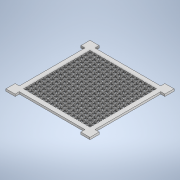
# Autodesk Inventor part: LED_Abstand
Saved by Autodesk Inventor 2022 (Build 260153000, 153)
## iProperties
Created: 2022-02-17
Part Number: LED_Abstand
Material: Generisch
Document SubType Name: Modeling
Designer: Max
Density: 1 g/cm^3
Appearance: Vorgabe
Author: Max
Autodesk Inventor part; units mm, degrees
(part 1 of 3)
ref_plane "YZ Plane" through (0, 0, 0) normal (1, 0, 0) x (0, 1, 0)
ref_plane "XZ Plane" through (0, 0, 0) normal (0, 1, 0) x (-1, 0, 0)
ref_plane "XY Plane" through (0, 0, 0) normal (0, 0, 1) x (1, 0, 0)
sketch "Skizze1" plane through (0, 0, 0) normal (0, 1, 0) x (-1, 0, 0)
  line L0 (-21.9, -21.9) -> (-28.1, -21.9)
  line L1 (-28.1, -21.9) -> (-28.1, -28.1)
  line L2 (-28.1, -28.1) -> (-21.9, -28.1)
  line L3 (-21.9, -28.1) -> (-21.9, -21.9)
  line L4 (-21.9, -31.9) -> (-28.1, -31.9)
  line L5 (-28.1, -31.9) -> (-28.1, -38.1)
  line L6 (-28.1, -38.1) -> (-21.9, -38.1)
  line L7 (-21.9, -38.1) -> (-21.9, -31.9)
  line L8 (-21.9, -41.9) -> (-28.1, -41.9)
  line L9 (-28.1, -41.9) -> (-28.1, -48.1)
  line L10 (-28.1, -48.1) -> (-21.9, -48.1)
  line L11 (-21.9, -48.1) -> (-21.9, -41.9)
  line L12 (-21.9, -51.9) -> (-28.1, -51.9)
  line L13 (-28.1, -51.9) -> (-28.1, -58.1)
  line L14 (-28.1, -58.1) -> (-21.9, -58.1)
  line L15 (-21.9, -58.1) -> (-21.9, -51.9)
  line L16 (-21.9, -61.9) -> (-28.1, -61.9)
  line L17 (-28.1, -61.9) -> (-28.1, -68.1)
  line L18 (-28.1, -68.1) -> (-21.9, -68.1)
  line L19 (-21.9, -68.1) -> (-21.9, -61.9)
  line L20 (-21.9, -28.1) -> (-21.9, -31.9) construction
  line L21 (-21.9, -38.1) -> (-21.9, -41.9) construction
  line L22 (-21.9, -48.1) -> (-21.9, -51.9) construction
  line L23 (-21.9, -58.1) -> (-21.9, -61.9) construction
  line L24 (-21.9, -21.9) -> (-21.9, -10) construction
  line L25 (-21.9, -21.9) -> (-10, -21.9) construction
  line L26 (-21.9, -71.9) -> (-28.1, -71.9)
  line L27 (-28.1, -71.9) -> (-28.1, -78.1)
  line L28 (-28.1, -78.1) -> (-21.9, -78.1)
  line L29 (-21.9, -78.1) -> (-21.9, -71.9)
  line L30 (-21.9, -81.9) -> (-28.1, -81.9)
  line L31 (-28.1, -81.9) -> (-28.1, -88.1)
  line L32 (-28.1, -88.1) -> (-21.9, -88.1)
  line L33 (-21.9, -88.1) -> (-21.9, -81.9)
  line L34 (-21.9, -91.9) -> (-28.1, -91.9)
  line L35 (-28.1, -91.9) -> (-28.1, -98.1)
  line L36 (-28.1, -98.1) -> (-21.9, -98.1)
  line L37 (-21.9, -98.1) -> (-21.9, -91.9)
  line L38 (-21.9, -101.9) -> (-28.1, -101.9)
  line L39 (-28.1, -101.9) -> (-28.1, -108.1)
  line L40 (-28.1, -108.1) -> (-21.9, -108.1)
  line L41 (-21.9, -108.1) -> (-21.9, -101.9)
  line L42 (-21.9, -111.9) -> (-28.1, -111.9)
  line L43 (-28.1, -111.9) -> (-28.1, -118.1)
  line L44 (-28.1, -118.1) -> (-21.9, -118.1)
  line L45 (-21.9, -118.1) -> (-21.9, -111.9)
  line L46 (-21.9, -78.1) -> (-21.9, -81.9) construction
  line L47 (-21.9, -88.1) -> (-21.9, -91.9) construction
  line L48 (-21.9, -98.1) -> (-21.9, -101.9) construction
  line L49 (-21.9, -108.1) -> (-21.9, -111.9) construction
  line L50 (-21.9, -68.1) -> (-21.9, -71.9) construction
  line L51 (-21.9, -121.9) -> (-28.1, -121.9)
  line L52 (-28.1, -121.9) -> (-28.1, -128.1)
  line L53 (-28.1, -128.1) -> (-21.9, -128.1)
  line L54 (-21.9, -128.1) -> (-21.9, -121.9)
  line L55 (-21.9, -131.9) -> (-28.1, -131.9)
  line L56 (-28.1, -131.9) -> (-28.1, -138.1)
  line L57 (-28.1, -138.1) -> (-21.9, -138.1)
  line L58 (-21.9, -138.1) -> (-21.9, -131.9)
  line L59 (-21.9, -141.9) -> (-28.1, -141.9)
  line L60 (-28.1, -141.9) -> (-28.1, -148.1)
  line L61 (-28.1, -148.1) -> (-21.9, -148.1)
  line L62 (-21.9, -148.1) -> (-21.9, -141.9)
  line L63 (-21.9, -151.9) -> (-28.1, -151.9)
  line L64 (-21.9, -138.1) -> (-21.9, -141.9) construction
  line L65 (-21.9, -148.1) -> (-21.9, -151.9) construction
  line L66 (-28.1, -151.9) -> (-28.1, -158.1)
  line L67 (-21.9, -158.1) -> (-21.9, -151.9)
  line L68 (-28.1, -158.1) -> (-21.9, -158.1)
  line L69 (-21.9, -128.1) -> (-21.9, -131.9) construction
  line L70 (-28.1, -178.1) -> (-21.9, -178.1)
  line L71 (-21.9, -171.9) -> (-28.1, -171.9)
  line L72 (-28.1, -171.9) -> (-28.1, -178.1)
  line L73 (-21.9, -178.1) -> (-21.9, -171.9)
  line L74 (-28.1, -168.1) -> (-21.9, -168.1)
  line L75 (-21.9, -168.1) -> (-21.9, -171.9) construction
  line L76 (-21.9, -161.9) -> (-28.1, -161.9)
  line L77 (-28.1, -161.9) -> (-28.1, -168.1)
  line L78 (-21.9, -168.1) -> (-21.9, -161.9)
  line L79 (-21.9, -158.1) -> (-21.9, -161.9) construction
  line L80 (-21.9, -118.1) -> (-21.9, -121.9) construction
  line L81 (-21.9, -178.1) -> (-21.9, -190) construction
  line L82 (-31.9, -21.9) -> (-38.1, -21.9)
  line L83 (-38.1, -21.9) -> (-38.1, -28.1)
  line L84 (-38.1, -28.1) -> (-31.9, -28.1)
  line L85 (-31.9, -28.1) -> (-31.9, -21.9)
  line L86 (-31.9, -31.9) -> (-38.1, -31.9)
  line L87 (-38.1, -31.9) -> (-38.1, -38.1)
  line L88 (-38.1, -38.1) -> (-31.9, -38.1)
  line L89 (-31.9, -38.1) -> (-31.9, -31.9)
  line L90 (-31.9, -41.9) -> (-38.1, -41.9)
  line L91 (-38.1, -41.9) -> (-38.1, -48.1)
  line L92 (-38.1, -48.1) -> (-31.9, -48.1)
  line L93 (-31.9, -48.1) -> (-31.9, -41.9)
  line L94 (-31.9, -51.9) -> (-38.1, -51.9)
  line L95 (-38.1, -51.9) -> (-38.1, -58.1)
  line L96 (-38.1, -58.1) -> (-31.9, -58.1)
  line L97 (-31.9, -58.1) -> (-31.9, -51.9)
  line L98 (-31.9, -61.9) -> (-38.1, -61.9)
  line L99 (-38.1, -61.9) -> (-38.1, -68.1)
  line L100 (-38.1, -68.1) -> (-31.9, -68.1)
  line L101 (-31.9, -68.1) -> (-31.9, -61.9)
  line L102 (-31.9, -28.1) -> (-31.9, -31.9) construction
  line L103 (-31.9, -38.1) -> (-31.9, -41.9) construction
  line L104 (-31.9, -48.1) -> (-31.9, -51.9) construction
  line L105 (-31.9, -58.1) -> (-31.9, -61.9) construction
  line L106 (-31.9, -71.9) -> (-38.1, -71.9)
  line L107 (-38.1, -71.9) -> (-38.1, -78.1)
  line L108 (-38.1, -78.1) -> (-31.9, -78.1)
  line L109 (-31.9, -78.1) -> (-31.9, -71.9)
  line L110 (-31.9, -81.9) -> (-38.1, -81.9)
  line L111 (-38.1, -81.9) -> (-38.1, -88.1)
  line L112 (-38.1, -88.1) -> (-31.9, -88.1)
  line L113 (-31.9, -88.1) -> (-31.9, -81.9)
  line L114 (-31.9, -91.9) -> (-38.1, -91.9)
  line L115 (-31.9, -78.1) -> (-31.9, -81.9) construction
  line L116 (-31.9, -88.1) -> (-31.9, -91.9) construction
  line L117 (-38.1, -91.9) -> (-38.1, -98.1)
  line L118 (-31.9, -98.1) -> (-31.9, -91.9)
  line L119 (-38.1, -98.1) -> (-31.9, -98.1)
  line L120 (-31.9, -98.1) -> (-31.9, -101.9) construction
  line L121 (-31.9, -101.9) -> (-38.1, -101.9)
  line L122 (-38.1, -101.9) -> (-38.1, -108.1)
  line L123 (-31.9, -108.1) -> (-31.9, -101.9)
  line L124 (-38.1, -108.1) -> (-31.9, -108.1)
  line L125 (-31.9, -111.9) -> (-38.1, -111.9)
  line L126 (-31.9, -108.1) -> (-31.9, -111.9) construction
  line L127 (-38.1, -118.1) -> (-31.9, -118.1)
  line L128 (-31.9, -118.1) -> (-31.9, -111.9)
  line L129 (-38.1, -111.9) -> (-38.1, -118.1)
  line L130 (-31.9, -68.1) -> (-31.9, -71.9) construction
  line L131 (-38.1, -158.1) -> (-31.9, -158.1)
  line L132 (-31.9, -151.9) -> (-38.1, -151.9)
  line L133 (-38.1, -151.9) -> (-38.1, -158.1)
  line L134 (-31.9, -158.1) -> (-31.9, -151.9)
  line L135 (-38.1, -148.1) -> (-31.9, -148.1)
  line L136 (-31.9, -148.1) -> (-31.9, -151.9) construction
  line L137 (-31.9, -121.9) -> (-38.1, -121.9)
  line L138 (-38.1, -121.9) -> (-38.1, -128.1)
  line L139 (-31.9, -128.1) -> (-31.9, -121.9)
  line L140 (-38.1, -128.1) -> (-31.9, -128.1)
  line L141 (-31.9, -128.1) -> (-31.9, -131.9) construction
  line L142 (-31.9, -131.9) -> (-38.1, -131.9)
  line L143 (-38.1, -131.9) -> (-38.1, -138.1)
  line L144 (-38.1, -138.1) -> (-31.9, -138.1)
  line L145 (-31.9, -138.1) -> (-31.9, -131.9)
  line L146 (-31.9, -141.9) -> (-38.1, -141.9)
  line L147 (-31.9, -138.1) -> (-31.9, -141.9) construction
  line L148 (-38.1, -141.9) -> (-38.1, -148.1)
  line L149 (-31.9, -148.1) -> (-31.9, -141.9)
  line L150 (-38.1, -178.1) -> (-31.9, -178.1)
  line L151 (-31.9, -161.9) -> (-38.1, -161.9)
  line L152 (-38.1, -161.9) -> (-38.1, -168.1)
  line L153 (-31.9, -168.1) -> (-31.9, -161.9)
  line L154 (-38.1, -168.1) -> (-31.9, -168.1)
  line L155 (-31.9, -168.1) -> (-31.9, -171.9) construction
  line L156 (-31.9, -171.9) -> (-38.1, -171.9)
  line L157 (-31.9, -178.1) -> (-31.9, -171.9)
  line L158 (-38.1, -171.9) -> (-38.1, -178.1)
  line L159 (-31.9, -158.1) -> (-31.9, -161.9) construction
  line L160 (-31.9, -118.1) -> (-31.9, -121.9) construction
  line L161 (-31.9, -21.9) -> (-28.1, -21.9) construction
  line L162 (-41.9, -21.9) -> (-48.1, -21.9)
  line L163 (-48.1, -21.9) -> (-48.1, -28.1)
  line L164 (-48.1, -28.1) -> (-41.9, -28.1)
  line L165 (-41.9, -28.1) -> (-41.9, -21.9)
  line L166 (-41.9, -31.9) -> (-48.1, -31.9)
  line L167 (-48.1, -31.9) -> (-48.1, -38.1)
  line L168 (-48.1, -38.1) -> (-41.9, -38.1)
  line L169 (-41.9, -38.1) -> (-41.9, -31.9)
  line L170 (-41.9, -41.9) -> (-48.1, -41.9)
  line L171 (-48.1, -41.9) -> (-48.1, -48.1)
  line L172 (-48.1, -48.1) -> (-41.9, -48.1)
  line L173 (-41.9, -48.1) -> (-41.9, -41.9)
  line L174 (-41.9, -51.9) -> (-48.1, -51.9)
  line L175 (-48.1, -51.9) -> (-48.1, -58.1)
  line L176 (-48.1, -58.1) -> (-41.9, -58.1)
  line L177 (-41.9, -58.1) -> (-41.9, -51.9)
  line L178 (-41.9, -61.9) -> (-48.1, -61.9)
  line L179 (-48.1, -61.9) -> (-48.1, -68.1)
  line L180 (-48.1, -68.1) -> (-41.9, -68.1)
  line L181 (-41.9, -68.1) -> (-41.9, -61.9)
  line L182 (-41.9, -28.1) -> (-41.9, -31.9) construction
  line L183 (-41.9, -38.1) -> (-41.9, -41.9) construction
  line L184 (-41.9, -48.1) -> (-41.9, -51.9) construction
  line L185 (-41.9, -58.1) -> (-41.9, -61.9) construction
  line L186 (-41.9, -21.9) -> (-38.1, -21.9) construction
  line L187 (-41.9, -71.9) -> (-48.1, -71.9)
  line L188 (-48.1, -71.9) -> (-48.1, -78.1)
  line L189 (-48.1, -78.1) -> (-41.9, -78.1)
  line L190 (-41.9, -78.1) -> (-41.9, -71.9)
  line L191 (-41.9, -81.9) -> (-48.1, -81.9)
  line L192 (-48.1, -81.9) -> (-48.1, -88.1)
  line L193 (-48.1, -88.1) -> (-41.9, -88.1)
  line L194 (-41.9, -88.1) -> (-41.9, -81.9)
  line L195 (-41.9, -91.9) -> (-48.1, -91.9)
  line L196 (-41.9, -78.1) -> (-41.9, -81.9) construction
  line L197 (-41.9, -88.1) -> (-41.9, -91.9) construction
  line L198 (-48.1, -91.9) -> (-48.1, -98.1)
  line L199 (-41.9, -98.1) -> (-41.9, -91.9)
  line L200 (-48.1, -98.1) -> (-41.9, -98.1)
  line L201 (-41.9, -98.1) -> (-41.9, -101.9) construction
  line L202 (-41.9, -101.9) -> (-48.1, -101.9)
  line L203 (-48.1, -101.9) -> (-48.1, -108.1)
  line L204 (-41.9, -108.1) -> (-41.9, -101.9)
  line L205 (-48.1, -108.1) -> (-41.9, -108.1)
  line L206 (-41.9, -111.9) -> (-48.1, -111.9)
  line L207 (-41.9, -108.1) -> (-41.9, -111.9) construction
  line L208 (-48.1, -118.1) -> (-41.9, -118.1)
  line L209 (-41.9, -118.1) -> (-41.9, -111.9)
  line L210 (-48.1, -111.9) -> (-48.1, -118.1)
  line L211 (-41.9, -68.1) -> (-41.9, -71.9) construction
  line L212 (-48.1, -158.1) -> (-41.9, -158.1)
  line L213 (-41.9, -151.9) -> (-48.1, -151.9)
  line L214 (-48.1, -151.9) -> (-48.1, -158.1)
  line L215 (-41.9, -158.1) -> (-41.9, -151.9)
  line L216 (-48.1, -148.1) -> (-41.9, -148.1)
  line L217 (-41.9, -148.1) -> (-41.9, -151.9) construction
  line L218 (-41.9, -121.9) -> (-48.1, -121.9)
  line L219 (-48.1, -121.9) -> (-48.1, -128.1)
  line L220 (-41.9, -128.1) -> (-41.9, -121.9)
  line L221 (-48.1, -128.1) -> (-41.9, -128.1)
  line L222 (-41.9, -128.1) -> (-41.9, -131.9) construction
  line L223 (-41.9, -131.9) -> (-48.1, -131.9)
  line L224 (-48.1, -131.9) -> (-48.1, -138.1)
  line L225 (-48.1, -138.1) -> (-41.9, -138.1)
  line L226 (-41.9, -138.1) -> (-41.9, -131.9)
  line L227 (-41.9, -141.9) -> (-48.1, -141.9)
  line L228 (-41.9, -138.1) -> (-41.9, -141.9) construction
  line L229 (-48.1, -141.9) -> (-48.1, -148.1)
  line L230 (-41.9, -148.1) -> (-41.9, -141.9)
  line L231 (-48.1, -178.1) -> (-41.9, -178.1)
  line L232 (-41.9, -161.9) -> (-48.1, -161.9)
  line L233 (-48.1, -161.9) -> (-48.1, -168.1)
  line L234 (-41.9, -168.1) -> (-41.9, -161.9)
  line L235 (-48.1, -168.1) -> (-41.9, -168.1)
  line L236 (-41.9, -168.1) -> (-41.9, -171.9) construction
  line L237 (-41.9, -171.9) -> (-48.1, -171.9)
  line L238 (-41.9, -178.1) -> (-41.9, -171.9)
  line L239 (-48.1, -171.9) -> (-48.1, -178.1)
  line L240 (-41.9, -158.1) -> (-41.9, -161.9) construction
  line L241 (-41.9, -118.1) -> (-41.9, -121.9) construction
  line L242 (-51.9, -81.9) -> (-58.1, -81.9)
  line L243 (-58.1, -88.1) -> (-51.9, -88.1)
  line L244 (-51.9, -88.1) -> (-51.9, -81.9)
  line L245 (-58.1, -81.9) -> (-58.1, -88.1)
  line L246 (-51.9, -78.1) -> (-51.9, -81.9) construction
  line L247 (-58.1, -78.1) -> (-51.9, -78.1)
  line L248 (-51.9, -91.9) -> (-58.1, -91.9)
  line L249 (-51.9, -88.1) -> (-51.9, -91.9) construction
  line L250 (-58.1, -98.1) -> (-51.9, -98.1)
  line L251 (-51.9, -98.1) -> (-51.9, -91.9)
  line L252 (-51.9, -98.1) -> (-51.9, -101.9) construction
  line L253 (-51.9, -108.1) -> (-51.9, -101.9)
  line L254 (-58.1, -101.9) -> (-58.1, -108.1)
  line L255 (-51.9, -108.1) -> (-51.9, -111.9) construction
  line L256 (-51.9, -101.9) -> (-58.1, -101.9)
  line L257 (-58.1, -108.1) -> (-51.9, -108.1)
  line L258 (-51.9, -48.1) -> (-51.9, -51.9) construction
  line L259 (-51.9, -51.9) -> (-58.1, -51.9)
  line L260 (-58.1, -51.9) -> (-58.1, -58.1)
  line L261 (-51.9, -58.1) -> (-51.9, -51.9)
  line L262 (-58.1, -58.1) -> (-51.9, -58.1)
  line L263 (-51.9, -58.1) -> (-51.9, -61.9) construction
  line L264 (-51.9, -61.9) -> (-58.1, -61.9)
  line L265 (-58.1, -61.9) -> (-58.1, -68.1)
  line L266 (-51.9, -68.1) -> (-51.9, -61.9)
  line L267 (-51.9, -71.9) -> (-58.1, -71.9)
  line L268 (-51.9, -68.1) -> (-51.9, -71.9) construction
  line L269 (-51.9, -78.1) -> (-51.9, -71.9)
  line L270 (-58.1, -71.9) -> (-58.1, -78.1)
  line L271 (-58.1, -68.1) -> (-51.9, -68.1)
  line L272 (-58.1, -91.9) -> (-58.1, -98.1)
  line L273 (-51.9, -21.9) -> (-58.1, -21.9)
  line L274 (-58.1, -21.9) -> (-58.1, -28.1)
  line L275 (-58.1, -28.1) -> (-51.9, -28.1)
  line L276 (-51.9, -28.1) -> (-51.9, -21.9)
  line L277 (-51.9, -31.9) -> (-58.1, -31.9)
  line L278 (-58.1, -31.9) -> (-58.1, -38.1)
  line L279 (-58.1, -38.1) -> (-51.9, -38.1)
  line L280 (-51.9, -38.1) -> (-51.9, -31.9)
  line L281 (-51.9, -41.9) -> (-58.1, -41.9)
  line L282 (-58.1, -41.9) -> (-58.1, -48.1)
  line L283 (-51.9, -48.1) -> (-51.9, -41.9)
  line L284 (-51.9, -38.1) -> (-51.9, -41.9) construction
  line L285 (-51.9, -28.1) -> (-51.9, -31.9) construction
  line L286 (-58.1, -48.1) -> (-51.9, -48.1)
  line L287 (-51.9, -111.9) -> (-58.1, -111.9)
  line L288 (-51.9, -118.1) -> (-51.9, -111.9)
  line L289 (-58.1, -111.9) -> (-58.1, -118.1)
  line L290 (-58.1, -118.1) -> (-51.9, -118.1)
  line L291 (-51.9, -121.9) -> (-58.1, -121.9)
  line L292 (-51.9, -128.1) -> (-51.9, -121.9)
  line L293 (-58.1, -128.1) -> (-51.9, -128.1)
  line L294 (-58.1, -121.9) -> (-58.1, -128.1)
  line L295 (-51.9, -131.9) -> (-58.1, -131.9)
  line L296 (-51.9, -128.1) -> (-51.9, -131.9) construction
  line L297 (-51.9, -118.1) -> (-51.9, -121.9) construction
  line L298 (-51.9, -161.9) -> (-58.1, -161.9)
  line L299 (-58.1, -161.9) -> (-58.1, -168.1)
  line L300 (-51.9, -168.1) -> (-51.9, -161.9)
  line L301 (-58.1, -168.1) -> (-51.9, -168.1)
  line L302 (-51.9, -168.1) -> (-51.9, -171.9) construction
  line L303 (-51.9, -171.9) -> (-58.1, -171.9)
  line L304 (-51.9, -178.1) -> (-51.9, -171.9)
  line L305 (-58.1, -171.9) -> (-58.1, -178.1)
  line L306 (-58.1, -178.1) -> (-51.9, -178.1)
  line L307 (-58.1, -158.1) -> (-51.9, -158.1)
  line L308 (-58.1, -138.1) -> (-51.9, -138.1)
  line L309 (-58.1, -131.9) -> (-58.1, -138.1)
  line L310 (-51.9, -141.9) -> (-58.1, -141.9)
  line L311 (-51.9, -138.1) -> (-51.9, -141.9) construction
  line L312 (-51.9, -148.1) -> (-51.9, -141.9)
  line L313 (-58.1, -148.1) -> (-51.9, -148.1)
  line L314 (-58.1, -141.9) -> (-58.1, -148.1)
  line L315 (-51.9, -148.1) -> (-51.9, -151.9) construction
  line L316 (-51.9, -151.9) -> (-58.1, -151.9)
  line L317 (-58.1, -151.9) -> (-58.1, -158.1)
  line L318 (-51.9, -158.1) -> (-51.9, -151.9)
  line L319 (-51.9, -158.1) -> (-51.9, -161.9) construction
  line L320 (-51.9, -138.1) -> (-51.9, -131.9)
  line L321 (-51.9, -21.9) -> (-48.1, -21.9) construction
  line L322 (-61.9, -21.9) -> (-68.1, -21.9)
  line L323 (-68.1, -21.9) -> (-68.1, -28.1)
  line L324 (-68.1, -28.1) -> (-61.9, -28.1)
  line L325 (-61.9, -28.1) -> (-61.9, -21.9)
  line L326 (-61.9, -31.9) -> (-68.1, -31.9)
  line L327 (-68.1, -31.9) -> (-68.1, -38.1)
  line L328 (-68.1, -38.1) -> (-61.9, -38.1)
  line L329 (-61.9, -38.1) -> (-61.9, -31.9)
  line L330 (-61.9, -41.9) -> (-68.1, -41.9)
  line L331 (-68.1, -41.9) -> (-68.1, -48.1)
  line L332 (-68.1, -48.1) -> (-61.9, -48.1)
  line L333 (-61.9, -48.1) -> (-61.9, -41.9)
  line L334 (-61.9, -51.9) -> (-68.1, -51.9)
  line L335 (-68.1, -51.9) -> (-68.1, -58.1)
  line L336 (-68.1, -58.1) -> (-61.9, -58.1)
  line L337 (-61.9, -58.1) -> (-61.9, -51.9)
  line L338 (-61.9, -61.9) -> (-68.1, -61.9)
  line L339 (-68.1, -61.9) -> (-68.1, -68.1)
  line L340 (-68.1, -68.1) -> (-61.9, -68.1)
  line L341 (-61.9, -68.1) -> (-61.9, -61.9)
  line L342 (-61.9, -28.1) -> (-61.9, -31.9) construction
  line L343 (-61.9, -38.1) -> (-61.9, -41.9) construction
  line L344 (-61.9, -48.1) -> (-61.9, -51.9) construction
  line L345 (-61.9, -58.1) -> (-61.9, -61.9) construction
  line L346 (-61.9, -21.9) -> (-58.1, -21.9) construction
  line L347 (-61.9, -71.9) -> (-68.1, -71.9)
  line L348 (-68.1, -71.9) -> (-68.1, -78.1)
  line L349 (-68.1, -78.1) -> (-61.9, -78.1)
  line L350 (-61.9, -78.1) -> (-61.9, -71.9)
  line L351 (-61.9, -81.9) -> (-68.1, -81.9)
  line L352 (-68.1, -81.9) -> (-68.1, -88.1)
  line L353 (-68.1, -88.1) -> (-61.9, -88.1)
  line L354 (-61.9, -88.1) -> (-61.9, -81.9)
  line L355 (-61.9, -91.9) -> (-68.1, -91.9)
  line L356 (-61.9, -78.1) -> (-61.9, -81.9) construction
  line L357 (-61.9, -88.1) -> (-61.9, -91.9) construction
  line L358 (-68.1, -91.9) -> (-68.1, -98.1)
  line L359 (-61.9, -98.1) -> (-61.9, -91.9)
  line L360 (-68.1, -98.1) -> (-61.9, -98.1)
  line L361 (-61.9, -98.1) -> (-61.9, -101.9) construction
  line L362 (-61.9, -101.9) -> (-68.1, -101.9)
  line L363 (-68.1, -101.9) -> (-68.1, -108.1)
  line L364 (-61.9, -108.1) -> (-61.9, -101.9)
  line L365 (-68.1, -108.1) -> (-61.9, -108.1)
  line L366 (-61.9, -111.9) -> (-68.1, -111.9)
  line L367 (-61.9, -108.1) -> (-61.9, -111.9) construction
  line L368 (-68.1, -118.1) -> (-61.9, -118.1)
  line L369 (-61.9, -118.1) -> (-61.9, -111.9)
  line L370 (-68.1, -111.9) -> (-68.1, -118.1)
  line L371 (-61.9, -68.1) -> (-61.9, -71.9) construction
  line L372 (-68.1, -158.1) -> (-61.9, -158.1)
  line L373 (-61.9, -151.9) -> (-68.1, -151.9)
  line L374 (-68.1, -151.9) -> (-68.1, -158.1)
  line L375 (-61.9, -158.1) -> (-61.9, -151.9)
  line L376 (-68.1, -148.1) -> (-61.9, -148.1)
  line L377 (-61.9, -148.1) -> (-61.9, -151.9) construction
  line L378 (-61.9, -121.9) -> (-68.1, -121.9)
  line L379 (-68.1, -121.9) -> (-68.1, -128.1)
  line L380 (-61.9, -128.1) -> (-61.9, -121.9)
  line L381 (-68.1, -128.1) -> (-61.9, -128.1)
  line L382 (-61.9, -128.1) -> (-61.9, -131.9) construction
  line L383 (-61.9, -131.9) -> (-68.1, -131.9)
  line L384 (-68.1, -131.9) -> (-68.1, -138.1)
  line L385 (-68.1, -138.1) -> (-61.9, -138.1)
  line L386 (-61.9, -138.1) -> (-61.9, -131.9)
  line L387 (-61.9, -141.9) -> (-68.1, -141.9)
  line L388 (-61.9, -138.1) -> (-61.9, -141.9) construction
  line L389 (-68.1, -141.9) -> (-68.1, -148.1)
  line L390 (-61.9, -148.1) -> (-61.9, -141.9)
  line L391 (-68.1, -178.1) -> (-61.9, -178.1)
  line L392 (-61.9, -161.9) -> (-68.1, -161.9)
  line L393 (-68.1, -161.9) -> (-68.1, -168.1)
  line L394 (-61.9, -168.1) -> (-61.9, -161.9)
  line L395 (-68.1, -168.1) -> (-61.9, -168.1)
  line L396 (-61.9, -168.1) -> (-61.9, -171.9) construction
  line L397 (-61.9, -171.9) -> (-68.1, -171.9)
  line L398 (-61.9, -178.1) -> (-61.9, -171.9)
  line L399 (-68.1, -171.9) -> (-68.1, -178.1)
  line L400 (-61.9, -158.1) -> (-61.9, -161.9) construction
  line L401 (-61.9, -118.1) -> (-61.9, -121.9) construction
  line L402 (-71.9, -81.9) -> (-78.1, -81.9)
  line L403 (-78.1, -88.1) -> (-71.9, -88.1)
  line L404 (-71.9, -88.1) -> (-71.9, -81.9)
  line L405 (-78.1, -81.9) -> (-78.1, -88.1)
  line L406 (-71.9, -78.1) -> (-71.9, -81.9) construction
  line L407 (-78.1, -78.1) -> (-71.9, -78.1)
  line L408 (-71.9, -91.9) -> (-78.1, -91.9)
  line L409 (-71.9, -88.1) -> (-71.9, -91.9) construction
  line L410 (-78.1, -98.1) -> (-71.9, -98.1)
  line L411 (-71.9, -98.1) -> (-71.9, -91.9)
  line L412 (-71.9, -98.1) -> (-71.9, -101.9) construction
  line L413 (-71.9, -108.1) -> (-71.9, -101.9)
  line L414 (-78.1, -101.9) -> (-78.1, -108.1)
  line L415 (-71.9, -108.1) -> (-71.9, -111.9) construction
  line L416 (-71.9, -101.9) -> (-78.1, -101.9)
  line L417 (-78.1, -108.1) -> (-71.9, -108.1)
  line L418 (-71.9, -48.1) -> (-71.9, -51.9) construction
  line L419 (-71.9, -51.9) -> (-78.1, -51.9)
  line L420 (-78.1, -51.9) -> (-78.1, -58.1)
  line L421 (-71.9, -58.1) -> (-71.9, -51.9)
  line L422 (-78.1, -58.1) -> (-71.9, -58.1)
  line L423 (-71.9, -58.1) -> (-71.9, -61.9) construction
  line L424 (-71.9, -61.9) -> (-78.1, -61.9)
  line L425 (-78.1, -61.9) -> (-78.1, -68.1)
  line L426 (-71.9, -68.1) -> (-71.9, -61.9)
  line L427 (-71.9, -71.9) -> (-78.1, -71.9)
  line L428 (-71.9, -68.1) -> (-71.9, -71.9) construction
  line L429 (-71.9, -78.1) -> (-71.9, -71.9)
  line L430 (-78.1, -71.9) -> (-78.1, -78.1)
  line L431 (-78.1, -68.1) -> (-71.9, -68.1)
  line L432 (-78.1, -91.9) -> (-78.1, -98.1)
  line L433 (-71.9, -21.9) -> (-78.1, -21.9)
  line L434 (-78.1, -21.9) -> (-78.1, -28.1)
  line L435 (-78.1, -28.1) -> (-71.9, -28.1)
  line L436 (-71.9, -28.1) -> (-71.9, -21.9)
  line L437 (-71.9, -31.9) -> (-78.1, -31.9)
  line L438 (-78.1, -31.9) -> (-78.1, -38.1)
  line L439 (-78.1, -38.1) -> (-71.9, -38.1)
  line L440 (-71.9, -38.1) -> (-71.9, -31.9)
  line L441 (-71.9, -41.9) -> (-78.1, -41.9)
  line L442 (-78.1, -41.9) -> (-78.1, -48.1)
  line L443 (-71.9, -48.1) -> (-71.9, -41.9)
  line L444 (-71.9, -38.1) -> (-71.9, -41.9) construction
  line L445 (-71.9, -28.1) -> (-71.9, -31.9) construction
  line L446 (-78.1, -48.1) -> (-71.9, -48.1)
  line L447 (-71.9, -111.9) -> (-78.1, -111.9)
  line L448 (-71.9, -118.1) -> (-71.9, -111.9)
  line L449 (-78.1, -111.9) -> (-78.1, -118.1)
  line L450 (-78.1, -118.1) -> (-71.9, -118.1)
  line L451 (-71.9, -121.9) -> (-78.1, -121.9)
  line L452 (-71.9, -128.1) -> (-71.9, -121.9)
  line L453 (-78.1, -128.1) -> (-71.9, -128.1)
  line L454 (-78.1, -121.9) -> (-78.1, -128.1)
  line L455 (-71.9, -131.9) -> (-78.1, -131.9)
  line L456 (-71.9, -128.1) -> (-71.9, -131.9) construction
  line L457 (-71.9, -118.1) -> (-71.9, -121.9) construction
  line L458 (-71.9, -161.9) -> (-78.1, -161.9)
  line L459 (-78.1, -161.9) -> (-78.1, -168.1)
  line L460 (-71.9, -168.1) -> (-71.9, -161.9)
  line L461 (-78.1, -168.1) -> (-71.9, -168.1)
  line L462 (-71.9, -168.1) -> (-71.9, -171.9) construction
  line L463 (-71.9, -171.9) -> (-78.1, -171.9)
  line L464 (-71.9, -178.1) -> (-71.9, -171.9)
  line L465 (-78.1, -171.9) -> (-78.1, -178.1)
  line L466 (-78.1, -178.1) -> (-71.9, -178.1)
  line L467 (-78.1, -158.1) -> (-71.9, -158.1)
  line L468 (-78.1, -138.1) -> (-71.9, -138.1)
  line L469 (-78.1, -131.9) -> (-78.1, -138.1)
  line L470 (-71.9, -141.9) -> (-78.1, -141.9)
  line L471 (-71.9, -138.1) -> (-71.9, -141.9) construction
  line L472 (-71.9, -148.1) -> (-71.9, -141.9)
  line L473 (-78.1, -148.1) -> (-71.9, -148.1)
  line L474 (-78.1, -141.9) -> (-78.1, -148.1)
  line L475 (-71.9, -148.1) -> (-71.9, -151.9) construction
  line L476 (-71.9, -151.9) -> (-78.1, -151.9)
  line L477 (-78.1, -151.9) -> (-78.1, -158.1)
  line L478 (-71.9, -158.1) -> (-71.9, -151.9)
  line L479 (-71.9, -158.1) -> (-71.9, -161.9) construction
  line L480 (-71.9, -138.1) -> (-71.9, -131.9)
  line L481 (-71.9, -21.9) -> (-68.1, -21.9) construction
  line L482 (-88.1, -21.9) -> (-88.1, -28.1)
  line L483 (-81.9, -31.9) -> (-88.1, -31.9)
  line L484 (-81.9, -28.1) -> (-81.9, -31.9) construction
  line L485 (-88.1, -28.1) -> (-81.9, -28.1)
  line L486 (-81.9, -21.9) -> (-88.1, -21.9)
  line L487 (-81.9, -28.1) -> (-81.9, -21.9)
  line L488 (-81.9, -21.9) -> (-78.1, -21.9) construction
  line L489 (-91.9, -21.9) -> (-88.1, -21.9) construction
  line L490 (-91.9, -28.1) -> (-91.9, -21.9)
  line L491 (-91.9, -21.9) -> (-98.1, -21.9)
  line L492 (-98.1, -21.9) -> (-98.1, -28.1)
  line L493 (-98.1, -28.1) -> (-91.9, -28.1)
  line L494 (-91.9, -28.1) -> (-91.9, -31.9) construction
  line L495 (-91.9, -31.9) -> (-98.1, -31.9)
  line L496 (-88.1, -48.1) -> (-81.9, -48.1)
  line L497 (-98.1, -58.1) -> (-91.9, -58.1)
  line L498 (-91.9, -51.9) -> (-98.1, -51.9)
  line L499 (-98.1, -51.9) -> (-98.1, -58.1)
  line L500 (-91.9, -58.1) -> (-91.9, -51.9)
  line L501 (-88.1, -51.9) -> (-88.1, -58.1)
  line L502 (-88.1, -58.1) -> (-81.9, -58.1)
  line L503 (-81.9, -58.1) -> (-81.9, -51.9)
  line L504 (-91.9, -48.1) -> (-91.9, -51.9) construction
  line L505 (-81.9, -51.9) -> (-88.1, -51.9)
  line L506 (-81.9, -48.1) -> (-81.9, -51.9) construction
  line L507 (-88.1, -31.9) -> (-88.1, -38.1)
  line L508 (-88.1, -38.1) -> (-81.9, -38.1)
  line L509 (-81.9, -38.1) -> (-81.9, -31.9)
  line L510 (-81.9, -41.9) -> (-88.1, -41.9)
  line L511 (-88.1, -41.9) -> (-88.1, -48.1)
  line L512 (-91.9, -38.1) -> (-91.9, -31.9)
  line L513 (-98.1, -31.9) -> (-98.1, -38.1)
  line L514 (-98.1, -38.1) -> (-91.9, -38.1)
  line L515 (-91.9, -38.1) -> (-91.9, -41.9) construction
  line L516 (-81.9, -38.1) -> (-81.9, -41.9) construction
  line L517 (-81.9, -48.1) -> (-81.9, -41.9)
  line L518 (-91.9, -41.9) -> (-98.1, -41.9)
  line L519 (-91.9, -48.1) -> (-91.9, -41.9)
  line L520 (-98.1, -48.1) -> (-91.9, -48.1)
  line L521 (-98.1, -41.9) -> (-98.1, -48.1)
  line L522 (-88.1, -68.1) -> (-81.9, -68.1)
  line L523 (-81.9, -71.9) -> (-88.1, -71.9)
  line L524 (-91.9, -71.9) -> (-98.1, -71.9)
  line L525 (-91.9, -68.1) -> (-91.9, -71.9) construction
  line L526 (-81.9, -68.1) -> (-81.9, -71.9) construction
  line L527 (-98.1, -78.1) -> (-91.9, -78.1)
  line L528 (-91.9, -78.1) -> (-91.9, -71.9)
  line L529 (-88.1, -71.9) -> (-88.1, -78.1)
  line L530 (-88.1, -78.1) -> (-81.9, -78.1)
  line L531 (-81.9, -78.1) -> (-81.9, -71.9)
  line L532 (-81.9, -78.1) -> (-81.9, -81.9) construction
  line L533 (-91.9, -78.1) -> (-91.9, -81.9) construction
  line L534 (-98.1, -71.9) -> (-98.1, -78.1)
  line L535 (-81.9, -88.1) -> (-81.9, -91.9) construction
  line L536 (-91.9, -88.1) -> (-91.9, -91.9) construction
  line L537 (-88.1, -88.1) -> (-81.9, -88.1)
  line L538 (-81.9, -81.9) -> (-88.1, -81.9)
  line L539 (-81.9, -88.1) -> (-81.9, -81.9)
  line L540 (-88.1, -81.9) -> (-88.1, -88.1)
  line L541 (-98.1, -88.1) -> (-91.9, -88.1)
  line L542 (-91.9, -81.9) -> (-98.1, -81.9)
  line L543 (-98.1, -81.9) -> (-98.1, -88.1)
  line L544 (-91.9, -88.1) -> (-91.9, -81.9)
  line L545 (-91.9, -108.1) -> (-91.9, -101.9)
  line L546 (-91.9, -108.1) -> (-91.9, -111.9) construction
  line L547 (-91.9, -118.1) -> (-91.9, -111.9)
  line L548 (-91.9, -101.9) -> (-98.1, -101.9)
  line L549 (-98.1, -101.9) -> (-98.1, -108.1)
  line L550 (-98.1, -108.1) -> (-91.9, -108.1)
  line L551 (-98.1, -111.9) -> (-98.1, -118.1)
  line L552 (-91.9, -111.9) -> (-98.1, -111.9)
  line L553 (-98.1, -118.1) -> (-91.9, -118.1)
  line L554 (-91.9, -141.9) -> (-98.1, -141.9)
  line L555 (-91.9, -148.1) -> (-91.9, -151.9) construction
  line L556 (-98.1, -141.9) -> (-98.1, -148.1)
  line L557 (-98.1, -148.1) -> (-91.9, -148.1)
  line L558 (-91.9, -158.1) -> (-91.9, -151.9)
  line L559 (-98.1, -158.1) -> (-91.9, -158.1)
  line L560 (-98.1, -151.9) -> (-98.1, -158.1)
  line L561 (-91.9, -151.9) -> (-98.1, -151.9)
  line L562 (-91.9, -148.1) -> (-91.9, -141.9)
  line L563 (-88.1, -131.9) -> (-88.1, -138.1)
  line L564 (-91.9, -131.9) -> (-98.1, -131.9)
  line L565 (-98.1, -138.1) -> (-91.9, -138.1)
  line L566 (-91.9, -138.1) -> (-91.9, -131.9)
  line L567 (-81.9, -138.1) -> (-81.9, -141.9) construction
  line L568 (-91.9, -138.1) -> (-91.9, -141.9) construction
  line L569 (-98.1, -131.9) -> (-98.1, -138.1)
  line L570 (-88.1, -151.9) -> (-88.1, -158.1)
  line L571 (-88.1, -141.9) -> (-88.1, -148.1)
  line L572 (-88.1, -158.1) -> (-81.9, -158.1)
  line L573 (-81.9, -158.1) -> (-81.9, -151.9)
  line L574 (-81.9, -151.9) -> (-88.1, -151.9)
  line L575 (-81.9, -148.1) -> (-81.9, -151.9) construction
  line L576 (-88.1, -148.1) -> (-81.9, -148.1)
  line L577 (-81.9, -148.1) -> (-81.9, -141.9)
  line L578 (-81.9, -141.9) -> (-88.1, -141.9)
  line L579 (-88.1, -111.9) -> (-88.1, -118.1)
  line L580 (-81.9, -111.9) -> (-88.1, -111.9)
  line L581 (-81.9, -118.1) -> (-81.9, -111.9)
  line L582 (-88.1, -101.9) -> (-88.1, -108.1)
  line L583 (-88.1, -108.1) -> (-81.9, -108.1)
  line L584 (-81.9, -108.1) -> (-81.9, -111.9) construction
  line L585 (-81.9, -101.9) -> (-88.1, -101.9)
  line L586 (-81.9, -108.1) -> (-81.9, -101.9)
  line L587 (-88.1, -118.1) -> (-81.9, -118.1)
  line L588 (-81.9, -121.9) -> (-88.1, -121.9)
  line L589 (-88.1, -121.9) -> (-88.1, -128.1)
  line L590 (-91.9, -128.1) -> (-91.9, -131.9) construction
  line L591 (-98.1, -128.1) -> (-91.9, -128.1)
  line L592 (-81.9, -131.9) -> (-88.1, -131.9)
  line L593 (-88.1, -138.1) -> (-81.9, -138.1)
  line L594 (-91.9, -121.9) -> (-98.1, -121.9)
  line L595 (-98.1, -121.9) -> (-98.1, -128.1)
  line L596 (-91.9, -128.1) -> (-91.9, -121.9)
  line L597 (-88.1, -128.1) -> (-81.9, -128.1)
  line L598 (-81.9, -128.1) -> (-81.9, -131.9) construction
  line L599 (-91.9, -118.1) -> (-91.9, -121.9) construction
  line L600 (-81.9, -128.1) -> (-81.9, -121.9)
  line L601 (-81.9, -118.1) -> (-81.9, -121.9) construction
  line L602 (-81.9, -138.1) -> (-81.9, -131.9)
  line L603 (-91.9, -91.9) -> (-98.1, -91.9)
  line L604 (-98.1, -98.1) -> (-91.9, -98.1)
  line L605 (-98.1, -91.9) -> (-98.1, -98.1)
  line L606 (-91.9, -98.1) -> (-91.9, -91.9)
  line L607 (-88.1, -91.9) -> (-88.1, -98.1)
  line L608 (-81.9, -91.9) -> (-88.1, -91.9)
  line L609 (-81.9, -98.1) -> (-81.9, -91.9)
  line L610 (-91.9, -98.1) -> (-91.9, -101.9) construction
  line L611 (-88.1, -98.1) -> (-81.9, -98.1)
  line L612 (-81.9, -98.1) -> (-81.9, -101.9) construction
  line L613 (-88.1, -178.1) -> (-81.9, -178.1)
  line L614 (-81.9, -161.9) -> (-88.1, -161.9)
  line L615 (-88.1, -161.9) -> (-88.1, -168.1)
  line L616 (-91.9, -161.9) -> (-98.1, -161.9)
  line L617 (-91.9, -158.1) -> (-91.9, -161.9) construction
  line L618 (-81.9, -158.1) -> (-81.9, -161.9) construction
  line L619 (-81.9, -168.1) -> (-81.9, -161.9)
  line L620 (-88.1, -168.1) -> (-81.9, -168.1)
  line L621 (-81.9, -168.1) -> (-81.9, -171.9) construction
  line L622 (-81.9, -171.9) -> (-88.1, -171.9)
  line L623 (-88.1, -171.9) -> (-88.1, -178.1)
  line L624 (-81.9, -178.1) -> (-81.9, -171.9)
  line L625 (-81.9, -58.1) -> (-81.9, -61.9) construction
  line L626 (-91.9, -58.1) -> (-91.9, -61.9) construction
  line L627 (-81.9, -61.9) -> (-88.1, -61.9)
  line L628 (-81.9, -68.1) -> (-81.9, -61.9)
  line L629 (-88.1, -61.9) -> (-88.1, -68.1)
  line L630 (-91.9, -61.9) -> (-98.1, -61.9)
  line L631 (-91.9, -68.1) -> (-91.9, -61.9)
  line L632 (-98.1, -61.9) -> (-98.1, -68.1)
  line L633 (-98.1, -68.1) -> (-91.9, -68.1)
  line L634 (-98.1, -161.9) -> (-98.1, -168.1)
  line L635 (-91.9, -168.1) -> (-91.9, -161.9)
  line L636 (-91.9, -168.1) -> (-91.9, -171.9) construction
  line L637 (-91.9, -171.9) -> (-98.1, -171.9)
  line L638 (-98.1, -171.9) -> (-98.1, -178.1)
  line L639 (-91.9, -178.1) -> (-91.9, -171.9)
  line L640 (-98.1, -178.1) -> (-91.9, -178.1)
  line L641 (-98.1, -168.1) -> (-91.9, -168.1)
  line L642 (-101.9, -21.9) -> (-108.1, -21.9)
  line L643 (-108.1, -21.9) -> (-108.1, -28.1)
  line L644 (-108.1, -28.1) -> (-101.9, -28.1)
  line L645 (-101.9, -28.1) -> (-101.9, -21.9)
  line L646 (-101.9, -31.9) -> (-108.1, -31.9)
  line L647 (-108.1, -31.9) -> (-108.1, -38.1)
  line L648 (-108.1, -38.1) -> (-101.9, -38.1)
  line L649 (-101.9, -38.1) -> (-101.9, -31.9)
  line L650 (-101.9, -41.9) -> (-108.1, -41.9)
  line L651 (-108.1, -41.9) -> (-108.1, -48.1)
  line L652 (-108.1, -48.1) -> (-101.9, -48.1)
  line L653 (-101.9, -48.1) -> (-101.9, -41.9)
  line L654 (-101.9, -51.9) -> (-108.1, -51.9)
  line L655 (-108.1, -51.9) -> (-108.1, -58.1)
  line L656 (-108.1, -58.1) -> (-101.9, -58.1)
  line L657 (-101.9, -58.1) -> (-101.9, -51.9)
  line L658 (-101.9, -61.9) -> (-108.1, -61.9)
  line L659 (-108.1, -61.9) -> (-108.1, -68.1)
  line L660 (-108.1, -68.1) -> (-101.9, -68.1)
  line L661 (-101.9, -68.1) -> (-101.9, -61.9)
  line L662 (-101.9, -28.1) -> (-101.9, -31.9) construction
  line L663 (-101.9, -38.1) -> (-101.9, -41.9) construction
  line L664 (-101.9, -48.1) -> (-101.9, -51.9) construction
  line L665 (-101.9, -58.1) -> (-101.9, -61.9) construction
  line L666 (-101.9, -21.9) -> (-98.1, -21.9) construction
  line L667 (-101.9, -71.9) -> (-108.1, -71.9)
  line L668 (-108.1, -71.9) -> (-108.1, -78.1)
  line L669 (-108.1, -78.1) -> (-101.9, -78.1)
  line L670 (-101.9, -78.1) -> (-101.9, -71.9)
  line L671 (-101.9, -81.9) -> (-108.1, -81.9)
  line L672 (-108.1, -81.9) -> (-108.1, -88.1)
  line L673 (-108.1, -88.1) -> (-101.9, -88.1)
  line L674 (-101.9, -88.1) -> (-101.9, -81.9)
  line L675 (-101.9, -91.9) -> (-108.1, -91.9)
  line L676 (-101.9, -78.1) -> (-101.9, -81.9) construction
  line L677 (-101.9, -88.1) -> (-101.9, -91.9) construction
  line L678 (-108.1, -91.9) -> (-108.1, -98.1)
  line L679 (-101.9, -98.1) -> (-101.9, -91.9)
  line L680 (-108.1, -98.1) -> (-101.9, -98.1)
  line L681 (-101.9, -98.1) -> (-101.9, -101.9) construction
  line L682 (-101.9, -101.9) -> (-108.1, -101.9)
  line L683 (-108.1, -101.9) -> (-108.1, -108.1)
  line L684 (-101.9, -108.1) -> (-101.9, -101.9)
  line L685 (-108.1, -108.1) -> (-101.9, -108.1)
  line L686 (-101.9, -111.9) -> (-108.1, -111.9)
  line L687 (-101.9, -108.1) -> (-101.9, -111.9) construction
  line L688 (-108.1, -118.1) -> (-101.9, -118.1)
  line L689 (-101.9, -118.1) -> (-101.9, -111.9)
  line L690 (-108.1, -111.9) -> (-108.1, -118.1)
  line L691 (-101.9, -68.1) -> (-101.9, -71.9) construction
  line L692 (-108.1, -158.1) -> (-101.9, -158.1)
  line L693 (-101.9, -151.9) -> (-108.1, -151.9)
  line L694 (-108.1, -151.9) -> (-108.1, -158.1)
  line L695 (-101.9, -158.1) -> (-101.9, -151.9)
  line L696 (-108.1, -148.1) -> (-101.9, -148.1)
  line L697 (-101.9, -148.1) -> (-101.9, -151.9) construction
  line L698 (-101.9, -121.9) -> (-108.1, -121.9)
  line L699 (-108.1, -121.9) -> (-108.1, -128.1)
  line L700 (-101.9, -128.1) -> (-101.9, -121.9)
  line L701 (-108.1, -128.1) -> (-101.9, -128.1)
  line L702 (-101.9, -128.1) -> (-101.9, -131.9) construction
  line L703 (-101.9, -131.9) -> (-108.1, -131.9)
  line L704 (-108.1, -131.9) -> (-108.1, -138.1)
  line L705 (-108.1, -138.1) -> (-101.9, -138.1)
  line L706 (-101.9, -138.1) -> (-101.9, -131.9)
  line L707 (-101.9, -141.9) -> (-108.1, -141.9)
  line L708 (-101.9, -138.1) -> (-101.9, -141.9) construction
  line L709 (-108.1, -141.9) -> (-108.1, -148.1)
  line L710 (-101.9, -148.1) -> (-101.9, -141.9)
  line L711 (-108.1, -178.1) -> (-101.9, -178.1)
  line L712 (-101.9, -161.9) -> (-108.1, -161.9)
  line L713 (-108.1, -161.9) -> (-108.1, -168.1)
  line L714 (-101.9, -168.1) -> (-101.9, -161.9)
  line L715 (-108.1, -168.1) -> (-101.9, -168.1)
  line L716 (-101.9, -168.1) -> (-101.9, -171.9) construction
  line L717 (-101.9, -171.9) -> (-108.1, -171.9)
  line L718 (-101.9, -178.1) -> (-101.9, -171.9)
  line L719 (-108.1, -171.9) -> (-108.1, -178.1)
  line L720 (-101.9, -158.1) -> (-101.9, -161.9) construction
  line L721 (-101.9, -118.1) -> (-101.9, -121.9) construction
  line L722 (-111.9, -81.9) -> (-118.1, -81.9)
  line L723 (-118.1, -88.1) -> (-111.9, -88.1)
  line L724 (-111.9, -88.1) -> (-111.9, -81.9)
  line L725 (-118.1, -81.9) -> (-118.1, -88.1)
  line L726 (-111.9, -78.1) -> (-111.9, -81.9) construction
  line L727 (-118.1, -78.1) -> (-111.9, -78.1)
  line L728 (-111.9, -91.9) -> (-118.1, -91.9)
  line L729 (-111.9, -88.1) -> (-111.9, -91.9) construction
  line L730 (-118.1, -98.1) -> (-111.9, -98.1)
  line L731 (-111.9, -98.1) -> (-111.9, -91.9)
  line L732 (-111.9, -98.1) -> (-111.9, -101.9) construction
  line L733 (-111.9, -108.1) -> (-111.9, -101.9)
  line L734 (-118.1, -101.9) -> (-118.1, -108.1)
  line L735 (-111.9, -108.1) -> (-111.9, -111.9) construction
  line L736 (-111.9, -101.9) -> (-118.1, -101.9)
  line L737 (-118.1, -108.1) -> (-111.9, -108.1)
  line L738 (-111.9, -48.1) -> (-111.9, -51.9) construction
  line L739 (-111.9, -51.9) -> (-118.1, -51.9)
  line L740 (-118.1, -51.9) -> (-118.1, -58.1)
  line L741 (-111.9, -58.1) -> (-111.9, -51.9)
  line L742 (-118.1, -58.1) -> (-111.9, -58.1)
  line L743 (-111.9, -58.1) -> (-111.9, -61.9) construction
  line L744 (-111.9, -61.9) -> (-118.1, -61.9)
  line L745 (-118.1, -61.9) -> (-118.1, -68.1)
  line L746 (-111.9, -68.1) -> (-111.9, -61.9)
  line L747 (-111.9, -71.9) -> (-118.1, -71.9)
  line L748 (-111.9, -68.1) -> (-111.9, -71.9) construction
  line L749 (-111.9, -78.1) -> (-111.9, -71.9)
  line L750 (-118.1, -71.9) -> (-118.1, -78.1)
  line L751 (-118.1, -68.1) -> (-111.9, -68.1)
  line L752 (-118.1, -91.9) -> (-118.1, -98.1)
  line L753 (-111.9, -21.9) -> (-118.1, -21.9)
  line L754 (-118.1, -21.9) -> (-118.1, -28.1)
  line L755 (-118.1, -28.1) -> (-111.9, -28.1)
  line L756 (-111.9, -28.1) -> (-111.9, -21.9)
  line L757 (-111.9, -31.9) -> (-118.1, -31.9)
  line L758 (-118.1, -31.9) -> (-118.1, -38.1)
  line L759 (-118.1, -38.1) -> (-111.9, -38.1)
  line L760 (-111.9, -38.1) -> (-111.9, -31.9)
  line L761 (-111.9, -41.9) -> (-118.1, -41.9)
  line L762 (-118.1, -41.9) -> (-118.1, -48.1)
  line L763 (-111.9, -48.1) -> (-111.9, -41.9)
  line L764 (-111.9, -38.1) -> (-111.9, -41.9) construction
  line L765 (-111.9, -28.1) -> (-111.9, -31.9) construction
  line L766 (-118.1, -48.1) -> (-111.9, -48.1)
  line L767 (-111.9, -111.9) -> (-118.1, -111.9)
  line L768 (-111.9, -118.1) -> (-111.9, -111.9)
  line L769 (-118.1, -111.9) -> (-118.1, -118.1)
  line L770 (-118.1, -118.1) -> (-111.9, -118.1)
  line L771 (-111.9, -121.9) -> (-118.1, -121.9)
  line L772 (-111.9, -128.1) -> (-111.9, -121.9)
  line L773 (-118.1, -128.1) -> (-111.9, -128.1)
  line L774 (-118.1, -121.9) -> (-118.1, -128.1)
  line L775 (-111.9, -131.9) -> (-118.1, -131.9)
  line L776 (-111.9, -128.1) -> (-111.9, -131.9) construction
  line L777 (-111.9, -118.1) -> (-111.9, -121.9) construction
  line L778 (-111.9, -161.9) -> (-118.1, -161.9)
  line L779 (-118.1, -161.9) -> (-118.1, -168.1)
  line L780 (-111.9, -168.1) -> (-111.9, -161.9)
  line L781 (-118.1, -168.1) -> (-111.9, -168.1)
  line L782 (-111.9, -168.1) -> (-111.9, -171.9) construction
  line L783 (-111.9, -171.9) -> (-118.1, -171.9)
  line L784 (-111.9, -178.1) -> (-111.9, -171.9)
  line L785 (-118.1, -171.9) -> (-118.1, -178.1)
  line L786 (-118.1, -178.1) -> (-111.9, -178.1)
  line L787 (-118.1, -158.1) -> (-111.9, -158.1)
  line L788 (-118.1, -138.1) -> (-111.9, -138.1)
  line L789 (-118.1, -131.9) -> (-118.1, -138.1)
  line L790 (-111.9, -141.9) -> (-118.1, -141.9)
  line L791 (-111.9, -138.1) -> (-111.9, -141.9) construction
  line L792 (-111.9, -148.1) -> (-111.9, -141.9)
  line L793 (-118.1, -148.1) -> (-111.9, -148.1)
  line L794 (-118.1, -141.9) -> (-118.1, -148.1)
  line L795 (-111.9, -148.1) -> (-111.9, -151.9) construction
  line L796 (-111.9, -151.9) -> (-118.1, -151.9)
  line L797 (-118.1, -151.9) -> (-118.1, -158.1)
  line L798 (-111.9, -158.1) -> (-111.9, -151.9)
  line L799 (-111.9, -158.1) -> (-111.9, -161.9) construction
  line L800 (-111.9, -138.1) -> (-111.9, -131.9)
  line L801 (-111.9, -21.9) -> (-108.1, -21.9) construction
  line L802 (-128.1, -21.9) -> (-128.1, -28.1)
  line L803 (-121.9, -31.9) -> (-128.1, -31.9)
  line L804 (-121.9, -28.1) -> (-121.9, -31.9) construction
  line L805 (-128.1, -28.1) -> (-121.9, -28.1)
  line L806 (-121.9, -21.9) -> (-128.1, -21.9)
  line L807 (-121.9, -28.1) -> (-121.9, -21.9)
  line L808 (-121.9, -21.9) -> (-118.1, -21.9) construction
  line L809 (-131.9, -21.9) -> (-128.1, -21.9) construction
  line L810 (-131.9, -28.1) -> (-131.9, -21.9)
  line L811 (-131.9, -21.9) -> (-138.1, -21.9)
  line L812 (-138.1, -21.9) -> (-138.1, -28.1)
  line L813 (-138.1, -28.1) -> (-131.9, -28.1)
  line L814 (-131.9, -28.1) -> (-131.9, -31.9) construction
  line L815 (-131.9, -31.9) -> (-138.1, -31.9)
  line L816 (-128.1, -48.1) -> (-121.9, -48.1)
  line L817 (-138.1, -58.1) -> (-131.9, -58.1)
  line L818 (-131.9, -51.9) -> (-138.1, -51.9)
  line L819 (-138.1, -51.9) -> (-138.1, -58.1)
  line L820 (-131.9, -58.1) -> (-131.9, -51.9)
  line L821 (-128.1, -51.9) -> (-128.1, -58.1)
  line L822 (-128.1, -58.1) -> (-121.9, -58.1)
  line L823 (-121.9, -58.1) -> (-121.9, -51.9)
  line L824 (-131.9, -48.1) -> (-131.9, -51.9) construction
  line L825 (-121.9, -51.9) -> (-128.1, -51.9)
  line L826 (-121.9, -48.1) -> (-121.9, -51.9) construction
  line L827 (-128.1, -31.9) -> (-128.1, -38.1)
  line L828 (-128.1, -38.1) -> (-121.9, -38.1)
  line L829 (-121.9, -38.1) -> (-121.9, -31.9)
  line L830 (-121.9, -41.9) -> (-128.1, -41.9)
  line L831 (-128.1, -41.9) -> (-128.1, -48.1)
  line L832 (-131.9, -38.1) -> (-131.9, -31.9)
  line L833 (-138.1, -31.9) -> (-138.1, -38.1)
  line L834 (-138.1, -38.1) -> (-131.9, -38.1)
  line L835 (-131.9, -38.1) -> (-131.9, -41.9) construction
  line L836 (-121.9, -38.1) -> (-121.9, -41.9) construction
  line L837 (-121.9, -48.1) -> (-121.9, -41.9)
  line L838 (-131.9, -41.9) -> (-138.1, -41.9)
  line L839 (-131.9, -48.1) -> (-131.9, -41.9)
  line L840 (-138.1, -48.1) -> (-131.9, -48.1)
  line L841 (-138.1, -41.9) -> (-138.1, -48.1)
  line L842 (-128.1, -68.1) -> (-121.9, -68.1)
  line L843 (-121.9, -71.9) -> (-128.1, -71.9)
  line L844 (-131.9, -71.9) -> (-138.1, -71.9)
  line L845 (-131.9, -68.1) -> (-131.9, -71.9) construction
  line L846 (-121.9, -68.1) -> (-121.9, -71.9) construction
  line L847 (-138.1, -78.1) -> (-131.9, -78.1)
  line L848 (-131.9, -78.1) -> (-131.9, -71.9)
  line L849 (-128.1, -71.9) -> (-128.1, -78.1)
  line L850 (-128.1, -78.1) -> (-121.9, -78.1)
  line L851 (-121.9, -78.1) -> (-121.9, -71.9)
  line L852 (-121.9, -78.1) -> (-121.9, -81.9) construction
  line L853 (-131.9, -78.1) -> (-131.9, -81.9) construction
  line L854 (-138.1, -71.9) -> (-138.1, -78.1)
  line L855 (-121.9, -88.1) -> (-121.9, -91.9) construction
  line L856 (-131.9, -88.1) -> (-131.9, -91.9) construction
  line L857 (-128.1, -88.1) -> (-121.9, -88.1)
  line L858 (-121.9, -81.9) -> (-128.1, -81.9)
  line L859 (-121.9, -88.1) -> (-121.9, -81.9)
  line L860 (-128.1, -81.9) -> (-128.1, -88.1)
  line L861 (-138.1, -88.1) -> (-131.9, -88.1)
  line L862 (-131.9, -81.9) -> (-138.1, -81.9)
  line L863 (-138.1, -81.9) -> (-138.1, -88.1)
  line L864 (-131.9, -88.1) -> (-131.9, -81.9)
  line L865 (-131.9, -108.1) -> (-131.9, -101.9)
  line L866 (-131.9, -108.1) -> (-131.9, -111.9) construction
  line L867 (-131.9, -118.1) -> (-131.9, -111.9)
  line L868 (-131.9, -101.9) -> (-138.1, -101.9)
  line L869 (-138.1, -101.9) -> (-138.1, -108.1)
  line L870 (-138.1, -108.1) -> (-131.9, -108.1)
  line L871 (-138.1, -111.9) -> (-138.1, -118.1)
  line L872 (-131.9, -111.9) -> (-138.1, -111.9)
  line L873 (-138.1, -118.1) -> (-131.9, -118.1)
  line L874 (-131.9, -141.9) -> (-138.1, -141.9)
  line L875 (-131.9, -148.1) -> (-131.9, -151.9) construction
  line L876 (-138.1, -141.9) -> (-138.1, -148.1)
  line L877 (-138.1, -148.1) -> (-131.9, -148.1)
  line L878 (-131.9, -158.1) -> (-131.9, -151.9)
  line L879 (-138.1, -158.1) -> (-131.9, -158.1)
  line L880 (-138.1, -151.9) -> (-138.1, -158.1)
  line L881 (-131.9, -151.9) -> (-138.1, -151.9)
  line L882 (-131.9, -148.1) -> (-131.9, -141.9)
  line L883 (-128.1, -131.9) -> (-128.1, -138.1)
  line L884 (-131.9, -131.9) -> (-138.1, -131.9)
  line L885 (-138.1, -138.1) -> (-131.9, -138.1)
  line L886 (-131.9, -138.1) -> (-131.9, -131.9)
  line L887 (-121.9, -138.1) -> (-121.9, -141.9) construction
  line L888 (-131.9, -138.1) -> (-131.9, -141.9) construction
  line L889 (-138.1, -131.9) -> (-138.1, -138.1)
  line L890 (-128.1, -151.9) -> (-128.1, -158.1)
  line L891 (-128.1, -141.9) -> (-128.1, -148.1)
  line L892 (-128.1, -158.1) -> (-121.9, -158.1)
  line L893 (-121.9, -158.1) -> (-121.9, -151.9)
  line L894 (-121.9, -151.9) -> (-128.1, -151.9)
  line L895 (-121.9, -148.1) -> (-121.9, -151.9) construction
  line L896 (-128.1, -148.1) -> (-121.9, -148.1)
  line L897 (-121.9, -148.1) -> (-121.9, -141.9)
  line L898 (-121.9, -141.9) -> (-128.1, -141.9)
  line L899 (-128.1, -111.9) -> (-128.1, -118.1)
  line L900 (-121.9, -111.9) -> (-128.1, -111.9)
  line L901 (-121.9, -118.1) -> (-121.9, -111.9)
  line L902 (-128.1, -101.9) -> (-128.1, -108.1)
  line L903 (-128.1, -108.1) -> (-121.9, -108.1)
  line L904 (-121.9, -108.1) -> (-121.9, -111.9) construction
  line L905 (-121.9, -101.9) -> (-128.1, -101.9)
  line L906 (-121.9, -108.1) -> (-121.9, -101.9)
  line L907 (-128.1, -118.1) -> (-121.9, -118.1)
  line L908 (-121.9, -121.9) -> (-128.1, -121.9)
  line L909 (-128.1, -121.9) -> (-128.1, -128.1)
  line L910 (-131.9, -128.1) -> (-131.9, -131.9) construction
  line L911 (-138.1, -128.1) -> (-131.9, -128.1)
  line L912 (-121.9, -131.9) -> (-128.1, -131.9)
  line L913 (-128.1, -138.1) -> (-121.9, -138.1)
  line L914 (-131.9, -121.9) -> (-138.1, -121.9)
  line L915 (-138.1, -121.9) -> (-138.1, -128.1)
  line L916 (-131.9, -128.1) -> (-131.9, -121.9)
  line L917 (-128.1, -128.1) -> (-121.9, -128.1)
  line L918 (-121.9, -128.1) -> (-121.9, -131.9) construction
  line L919 (-131.9, -118.1) -> (-131.9, -121.9) construction
  line L920 (-121.9, -128.1) -> (-121.9, -121.9)
  line L921 (-121.9, -118.1) -> (-121.9, -121.9) construction
  line L922 (-121.9, -138.1) -> (-121.9, -131.9)
  line L923 (-131.9, -91.9) -> (-138.1, -91.9)
  line L924 (-138.1, -98.1) -> (-131.9, -98.1)
  line L925 (-138.1, -91.9) -> (-138.1, -98.1)
  line L926 (-131.9, -98.1) -> (-131.9, -91.9)
  line L927 (-128.1, -91.9) -> (-128.1, -98.1)
  line L928 (-121.9, -91.9) -> (-128.1, -91.9)
  line L929 (-121.9, -98.1) -> (-121.9, -91.9)
  line L930 (-131.9, -98.1) -> (-131.9, -101.9) construction
  line L931 (-128.1, -98.1) -> (-121.9, -98.1)
  line L932 (-121.9, -98.1) -> (-121.9, -101.9) construction
  line L933 (-128.1, -178.1) -> (-121.9, -178.1)
  line L934 (-121.9, -161.9) -> (-128.1, -161.9)
  line L935 (-128.1, -161.9) -> (-128.1, -168.1)
  line L936 (-131.9, -161.9) -> (-138.1, -161.9)
  line L937 (-131.9, -158.1) -> (-131.9, -161.9) construction
  line L938 (-121.9, -158.1) -> (-121.9, -161.9) construction
  line L939 (-121.9, -168.1) -> (-121.9, -161.9)
  line L940 (-128.1, -168.1) -> (-121.9, -168.1)
  line L941 (-121.9, -168.1) -> (-121.9, -171.9) construction
  line L942 (-121.9, -171.9) -> (-128.1, -171.9)
  line L943 (-128.1, -171.9) -> (-128.1, -178.1)
  line L944 (-121.9, -178.1) -> (-121.9, -171.9)
  line L945 (-121.9, -58.1) -> (-121.9, -61.9) construction
  line L946 (-131.9, -58.1) -> (-131.9, -61.9) construction
  line L947 (-121.9, -61.9) -> (-128.1, -61.9)
  line L948 (-121.9, -68.1) -> (-121.9, -61.9)
  line L949 (-128.1, -61.9) -> (-128.1, -68.1)
  line L950 (-131.9, -61.9) -> (-138.1, -61.9)
  line L951 (-131.9, -68.1) -> (-131.9, -61.9)
  line L952 (-138.1, -61.9) -> (-138.1, -68.1)
  line L953 (-138.1, -68.1) -> (-131.9, -68.1)
  line L954 (-138.1, -161.9) -> (-138.1, -168.1)
  line L955 (-131.9, -168.1) -> (-131.9, -161.9)
  line L956 (-131.9, -168.1) -> (-131.9, -171.9) construction
  line L957 (-131.9, -171.9) -> (-138.1, -171.9)
  line L958 (-138.1, -171.9) -> (-138.1, -178.1)
  line L959 (-131.9, -178.1) -> (-131.9, -171.9)
  line L960 (-138.1, -178.1) -> (-131.9, -178.1)
  line L961 (-138.1, -168.1) -> (-131.9, -168.1)
  line L962 (-151.9, -28.1) -> (-151.9, -21.9)
  line L963 (-158.1, -28.1) -> (-151.9, -28.1)
  line L964 (-151.9, -21.9) -> (-158.1, -21.9)
  line L965 (-158.1, -21.9) -> (-158.1, -28.1)
  line L966 (-151.9, -28.1) -> (-151.9, -31.9) construction
  line L967 (-161.9, -21.9) -> (-158.1, -21.9) construction
  line L968 (-151.9, -38.1) -> (-151.9, -31.9)
  line L969 (-151.9, -31.9) -> (-158.1, -31.9)
  line L970 (-158.1, -38.1) -> (-151.9, -38.1)
  line L971 (-158.1, -31.9) -> (-158.1, -38.1)
  line L972 (-151.9, -21.9) -> (-148.1, -21.9) construction
  line L973 (-141.9, -28.1) -> (-141.9, -31.9) construction
  line L974 (-148.1, -21.9) -> (-148.1, -28.1)
  line L975 (-148.1, -28.1) -> (-141.9, -28.1)
  line L976 (-141.9, -21.9) -> (-148.1, -21.9)
  line L977 (-141.9, -28.1) -> (-141.9, -21.9)
  line L978 (-141.9, -21.9) -> (-138.1, -21.9) construction
  line L979 (-148.1, -58.1) -> (-141.9, -58.1)
  line L980 (-141.9, -58.1) -> (-141.9, -61.9) construction
  line L981 (-151.9, -58.1) -> (-151.9, -61.9) construction
  line L982 (-151.9, -61.9) -> (-158.1, -61.9)
  line L983 (-158.1, -61.9) -> (-158.1, -68.1)
  line L984 (-151.9, -68.1) -> (-151.9, -61.9)
  line L985 (-141.9, -61.9) -> (-148.1, -61.9)
  line L986 (-148.1, -68.1) -> (-141.9, -68.1)
  line L987 (-141.9, -68.1) -> (-141.9, -61.9)
  line L988 (-148.1, -61.9) -> (-148.1, -68.1)
  line L989 (-141.9, -41.9) -> (-148.1, -41.9)
  line L990 (-148.1, -41.9) -> (-148.1, -48.1)
  line L991 (-148.1, -48.1) -> (-141.9, -48.1)
  line L992 (-141.9, -51.9) -> (-148.1, -51.9)
  line L993 (-148.1, -51.9) -> (-148.1, -58.1)
  line L994 (-141.9, -58.1) -> (-141.9, -51.9)
  line L995 (-141.9, -48.1) -> (-141.9, -51.9) construction
  line L996 (-141.9, -48.1) -> (-141.9, -41.9)
  line L997 (-158.1, -58.1) -> (-151.9, -58.1)
  line L998 (-151.9, -58.1) -> (-151.9, -51.9)
  line L999 (-151.9, -51.9) -> (-158.1, -51.9)
  line L1000 (-158.1, -51.9) -> (-158.1, -58.1)
  line L1001 (-141.9, -101.9) -> (-148.1, -101.9)
  line L1002 (-158.1, -108.1) -> (-151.9, -108.1)